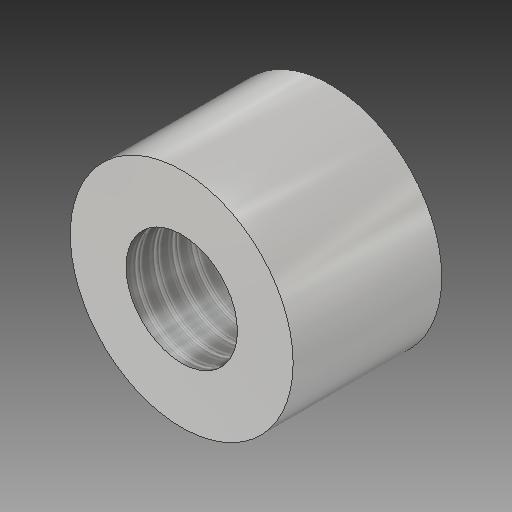
# Autodesk Inventor part: 中空Alスペーサー M3 L4
Saved by Autodesk Inventor 2017.3 (Build 213256000, 256)
## iProperties
Part Number: 中空Alスペーサー M3 L4
Material: アルミニウム
Document SubType Name: Modeling
Designer: 瑛飛
Mass: 0.229022 g
Surface Area: 1.55509 cm^2
Volume: 0.084823 cm^3
Density: 2.7 g/cm^3
Appearance: アルミニウム - つや出し
Author: 瑛飛
Autodesk Inventor part; units mm, degrees
ref_plane "YZ Plane" through (0, 0, 0) normal (1, 0, 0) x (0, 1, 0)
ref_plane "XZ Plane" through (0, 0, 0) normal (0, 1, 0) x (-1, 0, 0)
ref_plane "XY Plane" through (0, 0, 0) normal (0, 0, 1) x (1, 0, 0)
sketch "スケッチ1" plane through (0, 0, 0) normal (0, 0, 1) x (1, 0, 0)
  circle A0 centre (0, 0) radius 1.5
  circle A1 centre (0, 0) radius 3
  dimension "d0" = 3
  dimension "d1" = 6
  constraints: 2 centre point, 2 coincident
  measures "d0" diameter of A0
  measures "d1" diameter of A1
extrude "押し出し1" add sketch "スケッチ1" along normal blind 4
thread "ねじ1" size "M3x0.5" class "6H" standard "ANSI Metric M Profile" full length
equation "\"d1\" = 2 * d0"
